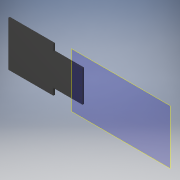
# Autodesk Inventor part: apriltag_calibration
Saved by Autodesk Inventor 2018 (Build 220112000, 112)
## iProperties
Created: 2018-12-11
Part Number: apriltag_calibration
Material: Generic
Document SubType Name: Modeling
Designer: jaspe
Density: 1 g/cm^3
Appearance: Default
Author: jaspe
Autodesk Inventor part; units mm, degrees
ref_plane "YZ Plane" through (0, 0, 0) normal (1, 0, 0) x (0, 1, 0)
ref_plane "XZ Plane" through (0, 0, 0) normal (0, 1, 0) x (-1, 0, 0)
ref_plane "XY Plane" through (0, 0, 0) normal (0, 0, 1) x (1, 0, 0)
ref_plane "Work Plane1" through (0, 0, -3) normal (0, 0, -1) x (-1, 0, 0)
sketch "Sketch3" plane through (0, 0, -3) normal (0, 0, -1) x (-1, 0, 0)
  circle A0 centre (45, -27) radius 1.5 projected
  circle A1 centre (72, 27) radius 1.5 projected
  circle A2 centre (18, 27) radius 1.5 projected
  circle A3 centre (18, -27) radius 1.5 projected
  circle A4 centre (90, 25) radius 1.25 projected
  circle A5 centre (90, -25) radius 1.25 projected
  circle A6 centre (90, 0) radius 1.25 projected
  circle A7 centre (63, 45) radius 2.5 projected
  circle A8 centre (63, -45) radius 2.5 projected
  circle A9 centre (-63, 45) radius 2.5 projected
  circle A10 centre (-90, 45) radius 2.5 projected
  circle A11 centre (90, -45) radius 2.5 projected
  circle A12 centre (90, 45) radius 2.5 projected
  circle A13 centre (-90, -45) radius 2.5 projected
  circle A14 centre (-63, -45) radius 2.5 projected
  circle A15 centre (-80, -5) radius 1.25 projected
  circle A16 centre (6, -5) radius 1.25 projected
  circle A17 centre (6, 35) radius 1.25 projected
  circle A18 centre (-80, 35) radius 1.25 projected
  circle A19 centre (-37, 35) radius 1.25 projected
  circle A20 centre (6, 15) radius 1.25 projected
  circle A21 centre (-37, -5) radius 1.25 projected
  circle A22 centre (-80, 15) radius 1.25 projected
  line L0 (100, 55) -> (-100, 55) projected
  line L1 (-100, 55) -> (-100, -55) projected
  line L2 (-100, -55) -> (100, -55) projected
  line L3 (100, -55) -> (100, 55) projected
  line L4 (115, 35) -> (85, 35)
  line L5 (85, 35) -> (85, -35)
  line L6 (85, -35) -> (115, -35)
  line L7 (115, -35) -> (115, 35)
  line L8 (115, 35) -> (85, -35) construction
  line L9 (85, 35) -> (115, -35) construction
  line L10 (100, 0) -> (200, 0)
  line L11 (100, 0) -> (200, 0) construction
  line L12 (250, 50) -> (150, 50)
  line L13 (150, 50) -> (150, -50)
  line L14 (150, -50) -> (250, -50)
  line L15 (250, -50) -> (250, 50)
  line L16 (250, 50) -> (150, -50) construction
  line L17 (150, 50) -> (250, -50) construction
  line L18 (185, 35) -> (115, 35)
  line L19 (115, 35) -> (115, -35)
  line L20 (115, -35) -> (185, -35)
  line L21 (185, -35) -> (185, 35)
  line L22 (185, 35) -> (115, -35) construction
  line L23 (115, 35) -> (185, -35) construction
  point P0 (0, 0)
  point P1 (150, 0)
  dimension "d0" = 30
  dimension "d1" = 70
  dimension "d2" = 100
  dimension "d3" = 0
  dimension "d4" = 100
  dimension "d5" = 100
  dimension "d6" = 70
  dimension "d7" = 70
  constraints: 40 end point, 8 midpoint, 6 parallel, 5 horizontal, 3 perpendicular, 1 collinear
  measures "d0" distance of L6.end L5.end
  measures "d1" distance of L5.end L4.end
  measures "d2" distance of L10.start L10.end
  measures "d3" distance between parallel lines of L10 L11
  measures "d4" distance of L14.end L13.end
  measures "d5" distance of L13.end L12.end
  measures "d6" distance of L20.end L6.end
  measures "d7" distance of L6.end L18.end
extrude "Extrusion1" add sketch "Sketch3" along normal blind 3 contours L4 L7 L10 L3 | L3 L6 L5 L4 | L10 L7 L6 L3 | L18 L13 L10 L7 | L10 L13 L20 L7 | L18 L21 L10 L13 | L13 L12 L15 L14 L20 L21 L18 | L10 L21 L20 L13
body "Solid1"
